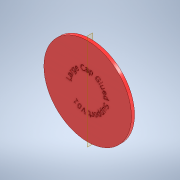
# Autodesk Inventor part: supportForLargeCap
Saved by Autodesk Inventor 2021.1 (Build 251245000, 245)
## iProperties
Created: 2020-09-25
Part Number: supportForLargeCap
Material: PC/ABS Plastic
Document SubType Name: Modeling
Designer: robst
Density: 0.357273 g/cm^3
Appearance: Light Red
Author: robst
Autodesk Inventor part; units mm, degrees
ref_plane "XZ Plane" through (0, 0, 0) normal (0, 1, 0) x (-1, 0, 0)
ref_plane "XY Plane" through (0, 0, 0) normal (0, 0, 1) x (1, 0, 0)
sketch "Sketch1" plane through (0, 0, 0) normal (0, 0, 1) x (1, 0, 0)
  circle A0 centre (0, 0) radius 88.9
  dimension "d0" = 177.8
  constraints: 1 centre point, 1 coincident
  measures "d0" diameter of A0
extrude "Extrusion1" add sketch "Sketch1" against normal blind 6.35
sketch "Sketch2" plane through (0, 0, 0) normal (0, 0, 1) x (1, 0, 0)
  circle A0 centre (0, 0) radius 38.1 construction
  line L0 (-32.4786, 6.8781) -> (-33.0946, 1.0235)
  line L1 (-33.0946, 1.0235) -> (-43.1988, 2.0867)
  line L2 (-43.1988, 2.0867) -> (-43.0575, 3.4296)
  line L3 (-43.0575, 3.4296) -> (-34.1488, 2.4922)
  line L4 (-34.1488, 2.4922) -> (-33.674, 7.0039)
  line L5 (-33.674, 7.0039) -> (-32.4786, 6.8781)
  spline S0 degree 2 poles (-31.6307, 12.0846) (-31.5706, 11.8998) (-31.3457, 11.2701) (-31.3063, 10.9968) knots 0 0 0 1 2 2 2
  spline S1 degree 2 poles (-31.3063, 10.9968) (-31.2407, 10.6193) (-31.2605, 9.958) (-31.442, 9.411) knots 0 0 0 1 2 2 2
  spline S2 degree 2 poles (-31.442, 9.411) (-31.5898, 8.9655) (-32.1928, 8.2721) (-32.5987, 8.0684) knots 0 0 0 1 2 2 2
  spline S3 degree 2 poles (-32.5987, 8.0684) (-32.9915, 7.8778) (-33.9834, 7.8165) (-34.4679, 7.9772) knots 0 0 0 1 2 2 2
  spline S4 degree 2 poles (-34.4679, 7.9772) (-35.2181, 8.2261) (-36.071, 9.2116) (-36.1476, 10.0004) knots 0 0 0 1 2 2 2
  spline S5 degree 2 poles (-36.1476, 10.0004) (-36.2267, 10.7033) (-35.8881, 12.4299) (-35.624, 13.4093) knots 0 0 0 1 2 2 2
  line L6 (-35.624, 13.4093) -> (-35.8584, 13.4871)
  spline S6 degree 2 poles (-35.8584, 13.4871) (-36.2804, 13.627) (-36.8895, 13.5429) (-37.1158, 13.3577) knots 0 0 0 1 2 2 2
  spline S7 degree 2 poles (-37.1158, 13.3577) (-37.342, 13.1725) (-37.6588, 12.5315) (-37.778, 12.1721) knots 0 0 0 1 2 2 2
  spline S8 degree 2 poles (-37.778, 12.1721) (-37.918, 11.7501) (-38.0464, 10.5262) (-37.9934, 9.8753) knots 0 0 0 1 2 2 2
  line L7 (-37.9934, 9.8753) -> (-38.0167, 9.805)
  line L8 (-38.0167, 9.805) -> (-39.2593, 10.2172)
  spline S9 degree 2 poles (-39.2593, 10.2172) (-39.2416, 10.5843) (-39.0586, 11.9203) (-38.8538, 12.5376) knots 0 0 0 1 2 2 2
  spline S10 degree 2 poles (-38.8538, 12.5376) (-38.605, 13.2878) (-38.0309, 14.2338) (-37.5914, 14.539) knots 0 0 0 1 2 2 2
  spline S11 degree 2 poles (-37.5914, 14.539) (-37.1622, 14.8391) (-36.087, 14.9161) (-35.4071, 14.6906) knots 0 0 0 1 2 2 2
  line L9 (-35.4071, 14.6906) -> (-30.4605, 13.0496)
  line L10 (-30.4605, 13.0496) -> (-30.8649, 11.8306)
  line L11 (-30.8649, 11.8306) -> (-31.6307, 12.0846)
  line L12 (-32.6466, 12.4216) -> (-34.655, 13.0878)
  spline S12 degree 2 poles (-34.655, 13.0878) (-34.7611, 12.6373) (-35.0663, 11.2725) (-35.0787, 10.8169) knots 0 0 0 1 2 2 2
  spline S13 degree 2 poles (-35.0787, 10.8169) (-35.0909, 10.2831) (-34.6836, 9.4453) (-34.1365, 9.2639) knots 0 0 0 1 2 2 2
  spline S14 degree 2 poles (-34.1365, 9.2639) (-33.5114, 9.0565) (-32.6451, 9.5498) (-32.4221, 10.2219) knots 0 0 0 1 2 2 2
  spline S15 degree 2 poles (-32.4221, 10.2219) (-32.2329, 10.7923) (-32.4141, 11.8934) (-32.6466, 12.4216) knots 0 0 0 1 2 2 2
  line L13 (-33.1361, 21.2152) -> (-33.1681, 21.1576)
  spline S16 degree 2 poles (-33.1681, 21.1576) (-33.276, 21.0481) (-33.4464, 20.7754) (-33.5543, 20.5811) knots 0 0 0 1 2 2 2
  spline S17 degree 2 poles (-33.5543, 20.5811) (-33.8062, 20.1276) (-33.9062, 19.0152) (-33.7414, 18.3963) knots 0 0 0 1 2 2 2
  line L14 (-33.7414, 18.3963) -> (-29.0128, 15.7693)
  line L15 (-29.0128, 15.7693) -> (-29.6365, 14.6465)
  line L16 (-29.6365, 14.6465) -> (-36.3013, 18.3491)
  line L17 (-36.3013, 18.3491) -> (-35.6775, 19.4718)
  line L18 (-35.6775, 19.4718) -> (-34.6843, 18.9201)
  spline S18 degree 2 poles (-34.6843, 18.9201) (-34.8914, 19.8357) (-34.8298, 20.9977) (-34.5899, 21.4295) knots 0 0 0 1 2 2 2
  spline S19 degree 2 poles (-34.5899, 21.4295) (-34.494, 21.6023) (-34.3836, 21.767) (-34.302, 21.863) knots 0 0 0 1 2 2 2
  line L19 (-34.302, 21.863) -> (-33.1361, 21.2152)
  spline S20 degree 2 poles (-26.0427, 18.4441) (-25.9138, 18.5077) (-25.4518, 18.7753) (-25.1883, 18.9733) knots 0 0 0 1 2 2 2
  spline S21 degree 2 poles (-25.1883, 18.9733) (-24.891, 19.1858) (-24.4221, 19.5767) (-24.1941, 19.8476) knots 0 0 0 1 2 2 2
  spline S22 degree 2 poles (-24.1941, 19.8476) (-23.8124, 20.3011) (-23.5216, 21.1325) (-23.5873, 21.4891) knots 0 0 0 1 2 2 2
  spline S23 degree 2 poles (-23.5873, 21.4891) (-23.6583, 21.8395) (-24.1076, 22.4436) (-24.4666, 22.7458) knots 0 0 0 1 2 2 2
  line L20 (-24.4666, 22.7458) -> (-24.9768, 23.1753)
  spline S24 degree 2 poles (-24.9768, 23.1753) (-24.9644, 22.4868) (-25.2784, 21.449) (-25.7609, 20.8757) knots 0 0 0 1 2 2 2
  spline S25 degree 2 poles (-25.7609, 20.8757) (-26.5986, 19.8805) (-29.0703, 19.9485) (-30.4624, 21.1202) knots 0 0 0 1 2 2 2
  spline S26 degree 2 poles (-30.4624, 21.1202) (-31.1868, 21.7299) (-31.9634, 23.0831) (-32.074, 23.7573) knots 0 0 0 1 2 2 2
  spline S27 degree 2 poles (-32.074, 23.7573) (-32.1699, 24.3977) (-31.8212, 25.6431) (-31.4182, 26.1218) knots 0 0 0 1 2 2 2
  spline S28 degree 2 poles (-31.4182, 26.1218) (-31.0365, 26.5753) (-30.2656, 27.0565) (-29.7893, 27.226) knots 0 0 0 1 2 2 2
  line L21 (-29.7893, 27.226) -> (-29.9873, 27.4894)
  line L22 (-29.9873, 27.4894) -> (-29.2079, 28.4154)
  line L23 (-29.2079, 28.4154) -> (-24.0427, 24.0678)
  spline S29 degree 2 poles (-24.0427, 24.0678) (-22.5561, 22.8166) (-22.2572, 20.3588) (-23.3759, 19.0297) knots 0 0 0 1 2 2 2
  spline S30 degree 2 poles (-23.3759, 19.0297) (-23.7364, 18.6014) (-24.6279, 17.8236) (-25.0647, 17.5347) knots 0 0 0 1 2 2 2
  line L24 (-25.0647, 17.5347) -> (-26.0851, 18.3937)
  line L25 (-26.0851, 18.3937) -> (-26.0427, 18.4441)
  line L26 (-25.7831, 23.8539) -> (-28.9894, 26.5526)
  spline S31 degree 2 poles (-28.9894, 26.5526) (-29.4732, 26.3357) (-30.144, 25.8457) (-30.4038, 25.537) knots 0 0 0 1 2 2 2
  spline S32 degree 2 poles (-30.4038, 25.537) (-31.0294, 24.7937) (-30.6544, 23.0145) (-29.6277, 22.1503) knots 0 0 0 1 2 2 2
  spline S33 degree 2 poles (-29.6277, 22.1503) (-28.6576, 21.3338) (-27.0974, 21.129) (-26.4824, 21.8597) knots 0 0 0 1 2 2 2
  spline S34 degree 2 poles (-26.4824, 21.8597) (-26.159, 22.2439) (-25.7827, 23.3047) (-25.7831, 23.8539) knots 0 0 0 1 2 2 2
  spline S35 degree 2 poles (-19.2664, 26.6093) (-20.7283, 25.5121) (-23.5656, 25.9458) (-24.7024, 27.4604) knots 0 0 0 1 2 2 2
  spline S36 degree 2 poles (-24.7024, 27.4604) (-25.8193, 28.9486) (-25.5833, 31.8847) (-24.3255, 32.8287) knots 0 0 0 1 2 2 2
  spline S37 degree 2 poles (-24.3255, 32.8287) (-23.7592, 33.2537) (-22.6363, 33.5818) (-22.0517, 33.475) knots 0 0 0 1 2 2 2
  spline S38 degree 2 poles (-22.0517, 33.475) (-21.4605, 33.3731) (-20.3553, 32.6275) (-19.8067, 31.8966) knots 0 0 0 1 2 2 2
  line L27 (-19.8067, 31.8966) -> (-19.3866, 31.3369)
  line L28 (-19.3866, 31.3369) -> (-23.6076, 28.1688)
  spline S39 degree 2 poles (-23.6076, 28.1688) (-22.8119, 27.1087) (-20.9, 26.7833) (-19.9517, 27.495) knots 0 0 0 1 2 2 2
  spline S40 degree 2 poles (-19.9517, 27.495) (-19.6159, 27.7471) (-19.0777, 28.3878) (-18.9032, 28.704) knots 0 0 0 1 2 2 2
  spline S41 degree 2 poles (-18.9032, 28.704) (-18.7255, 29.0433) (-18.5165, 29.5604) (-18.4705, 29.7597) knots 0 0 0 1 2 2 2
  line L29 (-18.4705, 29.7597) -> (-18.4112, 29.8042)
  line L30 (-18.4112, 29.8042) -> (-17.571, 28.6847)
  spline S42 degree 2 poles (-17.571, 28.6847) (-17.6945, 28.4789) (-18.0763, 27.8629) (-18.2425, 27.6454) knots 0 0 0 1 2 2 2
  spline S43 degree 2 poles (-18.2425, 27.6454) (-18.4746, 27.3374) (-18.8976, 26.8861) (-19.2664, 26.6093) knots 0 0 0 1 2 2 2
  spline S44 degree 2 poles (-20.9757, 31.3693) (-21.3002, 31.7742) (-21.9261, 32.2516) (-22.2439, 32.3321) knots 0 0 0 1 2 2 2
  spline S45 degree 2 poles (-22.2439, 32.3321) (-22.5947, 32.4292) (-23.3373, 32.2527) (-23.7522, 31.9413) knots 0 0 0 1 2 2 2
  spline S46 degree 2 poles (-23.7522, 31.9413) (-24.1604, 31.6349) (-24.5505, 30.9613) (-24.6096, 30.5463) knots 0 0 0 1 2 2 2
  spline S47 degree 2 poles (-24.6096, 30.5463) (-24.6572, 30.1297) (-24.4544, 29.3657) (-24.1957, 28.9525) knots 0 0 0 1 2 2 2
  line L31 (-24.1957, 28.9525) -> (-20.9757, 31.3693)
  spline S48 degree 2 poles (-8.1335, 31.8258) (-9.0845, 31.5578) (-10.8741, 31.7464) (-11.6414, 32.2231) knots 0 0 0 1 2 2 2
  spline S49 degree 2 poles (-11.6414, 32.2231) (-12.4065, 32.6919) (-13.5843, 34.4129) (-13.9327, 35.6492) knots 0 0 0 1 2 2 2
  spline S50 degree 2 poles (-13.9327, 35.6492) (-14.2788, 36.8776) (-14.1663, 38.8767) (-13.7618, 39.7177) knots 0 0 0 1 2 2 2
  spline S51 degree 2 poles (-13.7618, 39.7177) (-13.3607, 40.5407) (-11.9541, 41.6813) (-10.9635, 41.9604) knots 0 0 0 1 2 2 2
  spline S52 degree 2 poles (-10.9635, 41.9604) (-10.4722, 42.0988) (-9.5682, 42.1996) (-9.1724, 42.1913) knots 0 0 0 1 2 2 2
  spline S53 degree 2 poles (-9.1724, 42.1913) (-8.8264, 42.1776) (-8.086, 42.0698) (-7.7119, 41.987) knots 0 0 0 1 2 2 2
  line L32 (-7.7119, 41.987) -> (-7.2698, 40.4179)
  line L33 (-7.2698, 40.4179) -> (-7.3728, 40.3888)
  spline S54 degree 2 poles (-7.3728, 40.3888) (-7.5918, 40.4982) (-8.2558, 40.7901) (-8.7044, 40.8947) knots 0 0 0 1 2 2 2
  spline S55 degree 2 poles (-8.7044, 40.8947) (-9.1349, 40.9958) (-10.0882, 41.0095) (-10.6588, 40.8487) knots 0 0 0 1 2 2 2
  spline S56 degree 2 poles (-10.6588, 40.8487) (-11.2849, 40.6723) (-12.2571, 39.8423) (-12.5387, 39.2326) knots 0 0 0 1 2 2 2
  spline S57 degree 2 poles (-12.5387, 39.2326) (-12.8101, 38.6173) (-12.8433, 36.9741) (-12.5775, 36.0311) knots 0 0 0 1 2 2 2
  spline S58 degree 2 poles (-12.5775, 36.0311) (-12.2939, 35.0246) (-11.4019, 33.7106) (-10.8412, 33.3297) knots 0 0 0 1 2 2 2
  spline S59 degree 2 poles (-10.8412, 33.3297) (-10.2929, 32.9624) (-9.0529, 32.7814) (-8.4348, 32.9556) knots 0 0 0 1 2 2 2
  spline S60 degree 2 poles (-8.4348, 32.9556) (-7.8721, 33.1141) (-6.9914, 33.6617) (-6.677, 33.9727) knots 0 0 0 1 2 2 2
  spline S61 degree 2 poles (-6.677, 33.9727) (-6.3784, 34.2792) (-5.968, 34.8567) (-5.8599, 35.0497) knots 0 0 0 1 2 2 2
  line L34 (-5.8599, 35.0497) -> (-5.7648, 35.0765)
  line L35 (-5.7648, 35.0765) -> (-5.3271, 33.5233)
  spline S62 degree 2 poles (-5.3271, 33.5233) (-5.6096, 33.2812) (-6.102, 32.843) (-6.4705, 32.6023) knots 0 0 0 1 2 2 2
  spline S63 degree 2 poles (-6.4705, 32.6023) (-6.8582, 32.3391) (-7.5471, 31.991) (-8.1335, 31.8258) knots 0 0 0 1 2 2 2
  spline S64 degree 2 poles (0.2363, 33.8598) (0.0843, 33.7387) (-0.4267, 33.3075) (-0.6689, 33.1748) knots 0 0 0 1 2 2 2
  spline S65 degree 2 poles (-0.6689, 33.1748) (-0.9994, 32.9811) (-1.6258, 32.768) (-2.2018, 32.7463) knots 0 0 0 1 2 2 2
  spline S66 degree 2 poles (-2.2018, 32.7463) (-2.6707, 32.7286) (-3.5315, 33.0504) (-3.8645, 33.3592) knots 0 0 0 1 2 2 2
  spline S67 degree 2 poles (-3.8645, 33.3592) (-4.1807, 33.6604) (-4.5856, 34.568) (-4.6048, 35.0781) knots 0 0 0 1 2 2 2
  spline S68 degree 2 poles (-4.6048, 35.0781) (-4.6346, 35.8679) (-4.0103, 37.012) (-3.2984, 37.3601) knots 0 0 0 1 2 2 2
  spline S69 degree 2 poles (-3.2984, 37.3601) (-2.6678, 37.6805) (-0.9319, 37.9683) (0.0779, 38.064) knots 0 0 0 1 2 2 2
  line L36 (0.0779, 38.064) -> (0.0686, 38.3109)
  spline S70 degree 2 poles (0.0686, 38.3109) (0.0519, 38.7552) (-0.2404, 39.2962) (-0.4931, 39.4432) knots 0 0 0 1 2 2 2
  spline S71 degree 2 poles (-0.4931, 39.4432) (-0.7458, 39.5902) (-1.4571, 39.6623) (-1.8356, 39.648) knots 0 0 0 1 2 2 2
  spline S72 degree 2 poles (-1.8356, 39.648) (-2.2799, 39.6313) (-3.4712, 39.3228) (-4.0622, 39.0451) knots 0 0 0 1 2 2 2
  line L37 (-4.0622, 39.0451) -> (-4.1362, 39.0423)
  line L38 (-4.1362, 39.0423) -> (-4.1855, 40.3505)
  spline S73 degree 2 poles (-4.1855, 40.3505) (-3.8354, 40.4625) (-2.5201, 40.7593) (-1.8701, 40.7838) knots 0 0 0 1 2 2 2
  spline S74 degree 2 poles (-1.8701, 40.7838) (-1.0803, 40.8135) (0.0068, 40.6073) (0.4467, 40.3025) knots 0 0 0 1 2 2 2
  spline S75 degree 2 poles (0.4467, 40.3025) (0.8781, 40.0057) (1.327, 39.0257) (1.354, 38.3099) knots 0 0 0 1 2 2 2
  line L39 (1.354, 38.3099) -> (1.5502, 33.1018)
  line L40 (1.5502, 33.1018) -> (0.2667, 33.0535)
  line L41 (0.2667, 33.0535) -> (0.2363, 33.8598)
  line L42 (0.196, 34.9294) -> (0.1163, 37.0438)
  spline S76 degree 2 poles (0.1163, 37.0438) (-0.3428, 36.9853) (-1.728, 36.7931) (-2.1591, 36.645) knots 0 0 0 1 2 2 2
  spline S77 degree 2 poles (-2.1591, 36.645) (-2.6634, 36.4695) (-3.3053, 35.7944) (-3.2836, 35.2185) knots 0 0 0 1 2 2 2
  spline S78 degree 2 poles (-3.2836, 35.2185) (-3.2588, 34.5603) (-2.4932, 33.9217) (-1.7856, 33.9484) knots 0 0 0 1 2 2 2
  spline S79 degree 2 poles (-1.7856, 33.9484) (-1.185, 33.971) (-0.2173, 34.5265) (0.196, 34.9294) knots 0 0 0 1 2 2 2
  spline S80 degree 2 poles (10.3689, 35.7246) (10.0093, 33.8486) (7.7976, 31.9756) (6.431, 32.2375) knots 0 0 0 1 2 2 2
  spline S81 degree 2 poles (6.431, 32.2375) (5.873, 32.3445) (5.0655, 32.7675) (4.6719, 33.1196) knots 0 0 0 1 2 2 2
  line L43 (4.6719, 33.1196) -> (4.0705, 29.9822)
  line L44 (4.0705, 29.9822) -> (2.8091, 30.224)
  line L45 (2.8091, 30.224) -> (4.7729, 40.4692)
  line L46 (4.7729, 40.4692) -> (6.0344, 40.2274)
  line L47 (6.0344, 40.2274) -> (5.884, 39.443)
  spline S82 degree 2 poles (5.884, 39.443) (6.4352, 39.7817) (7.6919, 40.1276) (8.3631, 39.999) knots 0 0 0 1 2 2 2
  spline S83 degree 2 poles (8.3631, 39.999) (9.6488, 39.7525) (10.6975, 37.4389) (10.3689, 35.7246) knots 0 0 0 1 2 2 2
  spline S84 degree 2 poles (9.0391, 35.8286) (9.2856, 37.1143) (8.7401, 38.686) (7.8264, 38.8611) knots 0 0 0 1 2 2 2
  spline S85 degree 2 poles (7.8264, 38.8611) (7.2927, 38.9634) (6.1986, 38.6785) (5.6825, 38.3918) knots 0 0 0 1 2 2 2
  line L48 (5.6825, 38.3918) -> (4.8672, 34.1385)
  spline S86 degree 2 poles (4.8672, 34.1385) (5.3155, 33.8094) (5.9849, 33.4967) (6.4378, 33.4099) knots 0 0 0 1 2 2 2
  spline S87 degree 2 poles (6.4378, 33.4099) (7.4162, 33.2223) (8.7756, 34.454) (9.0391, 35.8286) knots 0 0 0 1 2 2 2
  spline S88 degree 2 poles (18.4556, 27.1493) (17.5523, 27.7387) (16.4159, 29.2666) (16.2424, 30.1761) knots 0 0 0 1 2 2 2
  spline S89 degree 2 poles (16.2424, 30.1761) (16.0735, 31.0924) (16.5899, 33.1345) (17.2963, 34.2171) knots 0 0 0 1 2 2 2
  spline S90 degree 2 poles (17.2963, 34.2171) (17.9666, 35.2446) (19.6076, 36.494) (20.5233, 36.7223) knots 0 0 0 1 2 2 2
  spline S91 degree 2 poles (20.5233, 36.7223) (21.4049, 36.9434) (23.3178, 36.5605) (24.2211, 35.9711) knots 0 0 0 1 2 2 2
  spline S92 degree 2 poles (24.2211, 35.9711) (24.6556, 35.6877) (25.3607, 35.0507) (25.6473, 34.7064) knots 0 0 0 1 2 2 2
  spline S93 degree 2 poles (25.6473, 34.7064) (25.8829, 34.4347) (26.3883, 33.6724) (26.53, 33.4226) knots 0 0 0 1 2 2 2
  line L49 (26.53, 33.4226) -> (25.6393, 32.0573)
  line L50 (25.6393, 32.0573) -> (25.5427, 32.1203)
  spline S94 degree 2 poles (25.5427, 32.1203) (25.4504, 32.4459) (25.2227, 33.0762) (24.9349, 33.5393) knots 0 0 0 1 2 2 2
  spline S95 degree 2 poles (24.9349, 33.5393) (24.7026, 33.9366) (23.9615, 34.7445) (23.4513, 35.0774) knots 0 0 0 1 2 2 2
  spline S96 degree 2 poles (23.4513, 35.0774) (22.2239, 35.8782) (19.5011, 35.02) (18.4979, 33.4823) knots 0 0 0 1 2 2 2
  spline S97 degree 2 poles (18.4979, 33.4823) (17.94, 32.6273) (17.5032, 31.0838) (17.5945, 30.395) knots 0 0 0 1 2 2 2
  spline S98 degree 2 poles (17.5945, 30.395) (17.672, 29.7152) (18.4049, 28.5784) (19.0531, 28.1555) knots 0 0 0 1 2 2 2
  spline S99 degree 2 poles (19.0531, 28.1555) (19.5289, 27.8451) (20.5704, 27.3621) (20.9845, 27.2886) knots 0 0 0 1 2 2 2
  line L51 (20.9845, 27.2886) -> (22.4197, 29.4883)
  line L52 (22.4197, 29.4883) -> (20.4475, 30.775)
  line L53 (20.4475, 30.775) -> (21.0954, 31.7679)
  line L54 (21.0954, 31.7679) -> (24.1846, 29.7524)
  line L55 (24.1846, 29.7524) -> (21.7597, 26.0357)
  spline S100 degree 2 poles (21.7597, 26.0357) (21.4829, 26.0786) (20.5585, 26.259) (20.1898, 26.3718) knots 0 0 0 1 2 2 2
  spline S101 degree 2 poles (20.1898, 26.3718) (19.6881, 26.5221) (18.9314, 26.8389) (18.4556, 27.1493) knots 0 0 0 1 2 2 2
  line L56 (23.3718, 23.3344) -> (22.4468, 24.2255)
  line L57 (22.4468, 24.2255) -> (29.8099, 31.8685)
  line L58 (29.8099, 31.8685) -> (30.7349, 30.9774)
  line L59 (30.7349, 30.9774) -> (23.3718, 23.3344)
  line L60 (28.2845, 17.2942) -> (27.5192, 18.3257)
  line L61 (27.5192, 18.3257) -> (28.1937, 18.8261)
  spline S102 degree 2 poles (28.1937, 18.8261) (27.4239, 18.9931) (26.3613, 19.5273) (25.9688, 20.0562) knots 0 0 0 1 2 2 2
  spline S103 degree 2 poles (25.9688, 20.0562) (25.6745, 20.453) (25.414, 21.3567) (25.507, 21.8255) knots 0 0 0 1 2 2 2
  spline S104 degree 2 poles (25.507, 21.8255) (25.5951, 22.301) (26.2455, 23.2346) (26.867, 23.6957) knots 0 0 0 1 2 2 2
  line L62 (26.867, 23.6957) -> (30.841, 26.6441)
  line L63 (30.841, 26.6441) -> (31.6063, 25.6126)
  line L64 (31.6063, 25.6126) -> (28.115, 23.0223)
  spline S105 degree 2 poles (28.115, 23.0223) (27.6257, 22.6593) (27.0383, 22.1107) (26.8935, 21.8085) knots 0 0 0 1 2 2 2
  spline S106 degree 2 poles (26.8935, 21.8085) (26.7486, 21.5062) (26.8493, 20.9145) (27.1486, 20.5112) knots 0 0 0 1 2 2 2
  spline S107 degree 2 poles (27.1486, 20.5112) (27.4282, 20.1343) (28.4908, 19.6002) (29.0665, 19.4737) knots 0 0 0 1 2 2 2
  line L65 (29.0665, 19.4737) -> (33.6422, 22.8685)
  line L66 (33.6422, 22.8685) -> (34.4075, 21.837)
  line L67 (34.4075, 21.837) -> (28.2845, 17.2942)
  spline S108 degree 2 poles (30.3491, 12.577) (29.6205, 14.2533) (30.6998, 16.913) (32.4365, 17.6679) knots 0 0 0 1 2 2 2
  spline S109 degree 2 poles (32.4365, 17.6679) (34.143, 18.4097) (36.9445, 17.4998) (37.5714, 16.0575) knots 0 0 0 1 2 2 2
  spline S110 degree 2 poles (37.5714, 16.0575) (37.8537, 15.4082) (37.9126, 14.2398) (37.6733, 13.6958) knots 0 0 0 1 2 2 2
  spline S111 degree 2 poles (37.6733, 13.6958) (37.4372, 13.1443) (36.4559, 12.242) (35.6177, 11.8776) knots 0 0 0 1 2 2 2
  line L68 (35.6177, 11.8776) -> (34.9759, 11.5987)
  line L69 (34.9759, 11.5987) -> (32.872, 16.4388)
  spline S112 degree 2 poles (32.872, 16.4388) (31.6563, 15.9103) (30.8968, 14.1258) (31.3695, 13.0385) knots 0 0 0 1 2 2 2
  spline S113 degree 2 poles (31.3695, 13.0385) (31.5368, 12.6534) (32.0355, 11.9814) (32.3027, 11.7384) knots 0 0 0 1 2 2 2
  spline S114 degree 2 poles (32.3027, 11.7384) (32.5915, 11.4869) (33.0462, 11.1639) (33.2294, 11.0729) knots 0 0 0 1 2 2 2
  line L70 (33.2294, 11.0729) -> (33.2589, 11.0049)
  line L71 (33.2589, 11.0049) -> (31.9752, 10.447)
  spline S115 degree 2 poles (31.9752, 10.447) (31.8036, 10.6147) (31.2928, 11.1289) (31.1198, 11.341) knots 0 0 0 1 2 2 2
  spline S116 degree 2 poles (31.1198, 11.341) (30.8739, 11.6381) (30.5329, 12.1542) (30.3491, 12.577) knots 0 0 0 1 2 2 2
  spline S117 degree 2 poles (35.3755, 13.137) (35.8447, 13.3589) (36.454, 13.8571) (36.6061, 14.1477) knots 0 0 0 1 2 2 2
  spline S118 degree 2 poles (36.6061, 14.1477) (36.7817, 14.4664) (36.7821, 15.2297) (36.5753, 15.7054) knots 0 0 0 1 2 2 2
  spline S119 degree 2 poles (36.5753, 15.7054) (36.3718, 16.1735) (35.8069, 16.709) (35.4169, 16.8627) knots 0 0 0 1 2 2 2
  spline S120 degree 2 poles (35.4169, 16.8627) (35.0227, 17.0055) (34.2325, 16.9853) (33.7706, 16.8294) knots 0 0 0 1 2 2 2
  line L72 (33.7706, 16.8294) -> (35.3755, 13.137)
  line L73 (33.0028, 3.1185) -> (32.7694, 4.3815)
  line L74 (32.7694, 4.3815) -> (33.5305, 4.5222)
  spline S121 degree 2 poles (33.5305, 4.5222) (33.2337, 4.7687) (32.8306, 5.138) (32.6391, 5.404) knots 0 0 0 1 2 2 2
  spline S122 degree 2 poles (32.6391, 5.404) (32.4601, 5.6473) (32.2163, 6.1967) (32.1459, 6.5772) knots 0 0 0 1 2 2 2
  spline S123 degree 2 poles (32.1459, 6.5772) (32.0322, 7.1925) (32.3508, 8.3231) (32.7773, 8.7787) knots 0 0 0 1 2 2 2
  spline S124 degree 2 poles (32.7773, 8.7787) (33.2039, 9.2343) (34.5864, 9.9084) (35.5336, 10.0835) knots 0 0 0 1 2 2 2
  spline S125 degree 2 poles (35.5336, 10.0835) (36.5214, 10.266) (38.0568, 10.0223) (38.6815, 9.6773) knots 0 0 0 1 2 2 2
  spline S126 degree 2 poles (38.6815, 9.6773) (39.2436, 9.3541) (40.0162, 8.2996) (40.1344, 7.66) knots 0 0 0 1 2 2 2
  spline S127 degree 2 poles (40.1344, 7.66) (40.2377, 7.1014) (40.1408, 6.2211) (39.967, 5.7117) knots 0 0 0 1 2 2 2
  line L75 (39.967, 5.7117) -> (43.2055, 6.3102)
  line L76 (43.2055, 6.3102) -> (43.4389, 5.0472)
  line L77 (43.4389, 5.0472) -> (33.0028, 3.1185)
  line L78 (34.5911, 4.7182) -> (38.9226, 5.5187)
  spline S128 degree 2 poles (38.9226, 5.5187) (39.0625, 6.0301) (39.0949, 6.8064) (39.0156, 7.2355) knots 0 0 0 1 2 2 2
  spline S129 degree 2 poles (39.0156, 7.2355) (38.836, 8.2071) (37.1752, 9.0389) (35.7988, 8.7845) knots 0 0 0 1 2 2 2
  spline S130 degree 2 poles (35.7988, 8.7845) (34.471, 8.5391) (33.226, 7.4382) (33.3981, 6.5072) knots 0 0 0 1 2 2 2
  spline S131 degree 2 poles (33.3981, 6.5072) (33.4893, 6.0133) (34.1283, 5.0931) (34.5911, 4.7182) knots 0 0 0 1 2 2 2
  spline S132 degree 2 poles (32.2963, -5.9446) (32.497, -4.8597) (33.2319, -3.4215) (33.6801, -2.8095) knots 0 0 0 1 2 2 2
  line L79 (33.6801, -2.8095) -> (35.3479, -3.1179)
  line L80 (35.3479, -3.1179) -> (35.3299, -3.2151)
  spline S133 degree 2 poles (35.3299, -3.2151) (34.5933, -3.7571) (33.6062, -5.291) (33.464, -6.0601) knots 0 0 0 1 2 2 2
  spline S134 degree 2 poles (33.464, -6.0601) (33.2603, -7.1611) (33.967, -8.4557) (34.7199, -8.595) knots 0 0 0 1 2 2 2
  spline S135 degree 2 poles (34.7199, -8.595) (35.319, -8.7058) (36.1732, -8.2526) (36.4777, -7.6474) knots 0 0 0 1 2 2 2
  spline S136 degree 2 poles (36.4777, -7.6474) (36.6926, -7.2099) (37.013, -6.4737) (37.265, -5.9259) knots 0 0 0 1 2 2 2
  spline S137 degree 2 poles (37.265, -5.9259) (37.4985, -5.4332) (38.0627, -4.6919) (38.453, -4.4375) knots 0 0 0 1 2 2 2
  spline S138 degree 2 poles (38.453, -4.4375) (38.8418, -4.1913) (39.7953, -4.016) (40.3782, -4.1238) knots 0 0 0 1 2 2 2
  spline S139 degree 2 poles (40.3782, -4.1238) (41.5926, -4.3484) (42.8857, -6.5469) (42.6146, -8.0123) knots 0 0 0 1 2 2 2
  spline S140 degree 2 poles (42.6146, -8.0123) (42.4589, -8.8543) (41.8514, -10.2825) (41.4174, -10.8637) knots 0 0 0 1 2 2 2
  line L81 (41.4174, -10.8637) -> (39.8305, -10.5702)
  line L82 (39.8305, -10.5702) -> (39.8485, -10.473)
  spline S141 degree 2 poles (39.8485, -10.473) (40.374, -10.0762) (41.2973, -8.7064) (41.4485, -7.8887) knots 0 0 0 1 2 2 2
  spline S142 degree 2 poles (41.4485, -7.8887) (41.6193, -6.9657) (40.9641, -5.6639) (40.2598, -5.5337) knots 0 0 0 1 2 2 2
  spline S143 degree 2 poles (40.2598, -5.5337) (39.6283, -5.4168) (38.751, -5.9495) (38.4642, -6.5496) knots 0 0 0 1 2 2 2
  spline S144 degree 2 poles (38.4642, -6.5496) (38.273, -6.9496) (37.7554, -8.1182) (37.5591, -8.5006) knots 0 0 0 1 2 2 2
  spline S145 degree 2 poles (37.5591, -8.5006) (37.0532, -9.4703) (35.6054, -10.1906) (34.6743, -10.0184) knots 0 0 0 1 2 2 2
  spline S146 degree 2 poles (34.6743, -10.0184) (34.0833, -9.909) (33.0382, -9.2217) (32.7209, -8.7192) knots 0 0 0 1 2 2 2
  spline S147 degree 2 poles (32.7209, -8.7192) (32.3721, -8.1607) (32.1271, -6.8594) (32.2963, -5.9446) knots 0 0 0 1 2 2 2
  line L83 (28.9807, -16.1005) -> (29.5016, -14.9265)
  line L84 (29.5016, -14.9265) -> (30.2692, -15.267)
  spline S148 degree 2 poles (30.2692, -15.267) (30.0355, -14.5148) (29.977, -13.3269) (30.2442, -12.7248) knots 0 0 0 1 2 2 2
  spline S149 degree 2 poles (30.2442, -12.7248) (30.4445, -12.2733) (31.1028, -11.6016) (31.5567, -11.4516) knots 0 0 0 1 2 2 2
  spline S150 degree 2 poles (31.5567, -11.4516) (32.0138, -11.2942) (33.1466, -11.4005) (33.8541, -11.7143) knots 0 0 0 1 2 2 2
  line L85 (33.8541, -11.7143) -> (38.3772, -13.7211)
  line L86 (38.3772, -13.7211) -> (37.8563, -14.8951)
  line L87 (37.8563, -14.8951) -> (33.8826, -13.1321)
  spline S151 degree 2 poles (33.8826, -13.1321) (33.3257, -12.885) (32.5589, -12.6439) (32.2245, -12.6667) knots 0 0 0 1 2 2 2
  spline S152 degree 2 poles (32.2245, -12.6667) (31.8902, -12.6895) (31.4248, -13.0685) (31.2211, -13.5276) knots 0 0 0 1 2 2 2
  spline S153 degree 2 poles (31.2211, -13.5276) (31.0308, -13.9566) (31.0892, -15.1444) (31.2626, -15.7078) knots 0 0 0 1 2 2 2
  line L88 (31.2626, -15.7078) -> (36.4706, -18.0184)
  line L89 (36.4706, -18.0184) -> (35.9497, -19.1924)
  line L90 (35.9497, -19.1924) -> (28.9807, -16.1005)
  spline S154 degree 2 poles (27.3575, -25.2057) (25.8385, -24.0476) (25.1477, -21.2329) (25.9913, -20.1263) knots 0 0 0 1 2 2 2
  spline S155 degree 2 poles (25.9913, -20.1263) (26.3357, -19.6746) (27.0744, -19.1403) (27.565, -18.9449) knots 0 0 0 1 2 2 2
  line L91 (27.565, -18.9449) -> (25.0246, -17.008)
  line L92 (25.0246, -17.008) -> (25.8033, -15.9866)
  line L93 (25.8033, -15.9866) -> (34.099, -22.3113)
  line L94 (34.099, -22.3113) -> (33.3203, -23.3327)
  line L95 (33.3203, -23.3327) -> (32.6852, -22.8485)
  spline S156 degree 2 poles (32.6852, -22.8485) (32.7427, -23.4928) (32.4922, -24.772) (32.0778, -25.3154) knots 0 0 0 1 2 2 2
  spline S157 degree 2 poles (32.0778, -25.3154) (31.2841, -26.3565) (28.7456, -26.264) (27.3575, -25.2057) knots 0 0 0 1 2 2 2
  spline S158 degree 2 poles (28.0434, -24.0617) (29.0844, -24.8554) (30.7344, -25.0677) (31.2985, -24.3278) knots 0 0 0 1 2 2 2
  spline S159 degree 2 poles (31.2985, -24.3278) (31.6279, -23.8957) (31.8606, -22.7893) (31.834, -22.1995) knots 0 0 0 1 2 2 2
  line L96 (31.834, -22.1995) -> (28.39, -19.5738)
  spline S160 degree 2 poles (28.39, -19.5738) (27.8956, -19.8285) (27.3173, -20.2883) (27.0377, -20.655) knots 0 0 0 1 2 2 2
  spline S161 degree 2 poles (27.0377, -20.655) (26.4337, -21.4472) (26.9303, -23.2131) (28.0434, -24.0617) knots 0 0 0 1 2 2 2
  spline S162 degree 2 poles (20.8036, -30.8379) (19.5928, -29.3605) (19.57, -26.4623) (20.6462, -25.5803) knots 0 0 0 1 2 2 2
  spline S163 degree 2 poles (20.6462, -25.5803) (21.0856, -25.2201) (21.9276, -24.8707) (22.4501, -24.7938) knots 0 0 0 1 2 2 2
  line L97 (22.4501, -24.7938) -> (20.4251, -22.3231)
  line L98 (20.4251, -22.3231) -> (21.4184, -21.5089)
  line L99 (21.4184, -21.5089) -> (28.031, -29.577)
  line L100 (28.031, -29.577) -> (27.0377, -30.3911)
  line L101 (27.0377, -30.3911) -> (26.5314, -29.7735)
  spline S164 degree 2 poles (26.5314, -29.7735) (26.4387, -30.4137) (25.8998, -31.6005) (25.3712, -32.0337) knots 0 0 0 1 2 2 2
  spline S165 degree 2 poles (25.3712, -32.0337) (24.3588, -32.8635) (21.9101, -32.1878) (20.8036, -30.8379) knots 0 0 0 1 2 2 2
  spline S166 degree 2 poles (21.7349, -29.883) (22.5647, -30.8954) (24.1212, -31.4827) (24.8408, -30.8929) knots 0 0 0 1 2 2 2
  spline S167 degree 2 poles (24.8408, -30.8929) (25.2611, -30.5485) (25.7428, -29.5256) (25.8529, -28.9456) knots 0 0 0 1 2 2 2
  line L102 (25.8529, -28.9456) -> (23.1077, -25.5961)
  spline S168 degree 2 poles (23.1077, -25.5961) (22.5679, -25.7298) (21.8991, -26.0438) (21.5425, -26.3361) knots 0 0 0 1 2 2 2
  spline S169 degree 2 poles (21.5425, -26.3361) (20.7719, -26.9676) (20.8476, -28.8004) (21.7349, -29.883) knots 0 0 0 1 2 2 2
  spline S170 degree 2 poles (13.1572, -34.5699) (12.3091, -32.84) (13.0482, -30.1394) (14.4381, -29.458) knots 0 0 0 1 2 2 2
  spline S171 degree 2 poles (14.4381, -29.458) (15.8648, -28.7584) (18.4519, -29.9017) (19.271, -31.5725) knots 0 0 0 1 2 2 2
  spline S172 degree 2 poles (19.271, -31.5725) (20.1119, -33.2876) (19.3578, -36.0139) (17.9828, -36.688) knots 0 0 0 1 2 2 2
  spline S173 degree 2 poles (17.9828, -36.688) (16.593, -37.3694) (14.0018, -36.2924) (13.1572, -34.5699) knots 0 0 0 1 2 2 2
  spline S174 degree 2 poles (14.3475, -33.9864) (14.9999, -35.317) (16.6026, -36.136) (17.4971, -35.6974) knots 0 0 0 1 2 2 2
  spline S175 degree 2 poles (17.4971, -35.6974) (18.3916, -35.2588) (18.7332, -33.4867) (18.0808, -32.156) knots 0 0 0 1 2 2 2
  spline S176 degree 2 poles (18.0808, -32.156) (17.4465, -30.8623) (15.8183, -30.01) (14.9237, -30.4486) knots 0 0 0 1 2 2 2
  spline S177 degree 2 poles (14.9237, -30.4486) (14.0366, -30.8835) (13.7023, -32.6705) (14.3475, -33.9864) knots 0 0 0 1 2 2 2
  line L103 (7.9312, -38.5381) -> (7.9947, -38.5208)
  spline S178 degree 2 poles (7.9947, -38.5208) (8.1485, -38.5216) (8.4627, -38.4533) (8.6772, -38.395) knots 0 0 0 1 2 2 2
  spline S179 degree 2 poles (8.6772, -38.395) (9.1778, -38.259) (10.0442, -37.5542) (10.3725, -37.0043) knots 0 0 0 1 2 2 2
  line L104 (10.3725, -37.0043) -> (8.9539, -31.7843)
  line L105 (8.9539, -31.7843) -> (10.1933, -31.4474)
  line L106 (10.1933, -31.4474) -> (12.1929, -38.8047)
  line L107 (12.1929, -38.8047) -> (10.9534, -39.1415)
  line L108 (10.9534, -39.1415) -> (10.6554, -38.0451)
  spline S180 degree 2 poles (10.6554, -38.0451) (10.1442, -38.8325) (9.269, -39.5993) (8.7923, -39.7289) knots 0 0 0 1 2 2 2
  spline S181 degree 2 poles (8.7923, -39.7289) (8.6016, -39.7807) (8.4066, -39.8166) (8.281, -39.8252) knots 0 0 0 1 2 2 2
  line L109 (8.281, -39.8252) -> (7.9312, -38.5381)
  spline S182 degree 2 poles (2.9956, -32.7473) (4.0339, -32.6237) (5.3442, -33.6699) (5.4971, -34.9535) knots 0 0 0 1 2 2 2
  line L110 (5.4971, -34.9535) -> (5.9965, -39.1476)
  line L111 (5.9965, -39.1476) -> (6.8549, -39.0454)
  line L112 (6.8549, -39.0454) -> (6.9805, -40.1)
  line L113 (6.9805, -40.1) -> (6.1221, -40.2023)
  line L114 (6.1221, -40.2023) -> (6.381, -42.377)
  line L115 (6.381, -42.377) -> (5.1056, -42.5288)
  line L116 (5.1056, -42.5288) -> (4.8467, -40.3541)
  line L117 (4.8467, -40.3541) -> (2.5003, -40.6335)
  line L118 (2.5003, -40.6335) -> (2.3747, -39.5789)
  line L119 (2.3747, -39.5789) -> (4.7211, -39.2995)
  line L120 (4.7211, -39.2995) -> (4.2918, -35.694)
  spline S183 degree 2 poles (4.2918, -35.694) (4.2236, -35.1217) (4.1078, -34.4971) (3.9367, -34.2438) knots 0 0 0 1 2 2 2
  spline S184 degree 2 poles (3.9367, -34.2438) (3.794, -34.0204) (3.2507, -33.8446) (2.8092, -33.8972) knots 0 0 0 1 2 2 2
  spline S185 degree 2 poles (2.8092, -33.8972) (2.4985, -33.9342) (1.9404, -34.1913) (1.8164, -34.2641) knots 0 0 0 1 2 2 2
  line L121 (1.8164, -34.2641) -> (1.7429, -34.2729)
  line L122 (1.7429, -34.2729) -> (1.6066, -33.1283)
  spline S186 degree 2 poles (1.6066, -33.1283) (1.9546, -32.9874) (2.6768, -32.7853) (2.9956, -32.7473) knots 0 0 0 1 2 2 2
  line L123 (-13.1413, -41.3426) -> (-7.5874, -32.1435)
  line L124 (-7.5874, -32.1435) -> (-6.1625, -32.4494)
  line L125 (-6.1625, -32.4494) -> (-4.874, -43.1175)
  line L126 (-4.874, -43.1175) -> (-6.2908, -42.8134)
  line L127 (-6.2908, -42.8134) -> (-7.2724, -33.9711)
  line L128 (-7.2724, -33.9711) -> (-11.797, -41.6312)
  line L129 (-11.797, -41.6312) -> (-13.1413, -41.3426)
  spline S187 degree 2 poles (-19.6245, -32.8187) (-18.4262, -30.3618) (-15.8755, -28.757) (-14.3881, -29.4824) knots 0 0 0 1 2 2 2
  spline S188 degree 2 poles (-14.3881, -29.4824) (-12.8785, -30.2187) (-12.6091, -33.2539) (-13.7821, -35.6589) knots 0 0 0 1 2 2 2
  spline S189 degree 2 poles (-13.7821, -35.6589) (-14.9876, -38.1306) (-17.531, -39.7207) (-19.0259, -38.9916) knots 0 0 0 1 2 2 2
  spline S190 degree 2 poles (-19.0259, -38.9916) (-20.5281, -38.259) (-20.7866, -35.2016) (-19.6245, -32.8187) knots 0 0 0 1 2 2 2
  spline S191 degree 2 poles (-16.6986, -30.8014) (-17.0963, -31.1662) (-17.9229, -32.4852) (-18.3812, -33.425) knots 0 0 0 1 2 2 2
  spline S192 degree 2 poles (-18.3812, -33.425) (-18.8396, -34.3649) (-19.3665, -35.8209) (-19.4089, -36.3773) knots 0 0 0 1 2 2 2
  spline S193 degree 2 poles (-19.4089, -36.3773) (-19.4513, -36.9338) (-19.042, -37.7288) (-18.5314, -37.9778) knots 0 0 0 1 2 2 2
  spline S194 degree 2 poles (-18.5314, -37.9778) (-18.0208, -38.2268) (-17.1276, -38.067) (-16.7006, -37.6799) knots 0 0 0 1 2 2 2
  spline S195 degree 2 poles (-16.7006, -37.6799) (-16.2882, -37.3039) (-15.4621, -35.948) (-15.0253, -35.0526) knots 0 0 0 1 2 2 2
  spline S196 degree 2 poles (-15.0253, -35.0526) (-14.5562, -34.0906) (-14.0466, -32.7452) (-13.9935, -32.1481) knots 0 0 0 1 2 2 2
  spline S197 degree 2 poles (-13.9935, -32.1481) (-13.9402, -31.5879) (-14.3497, -30.7561) (-14.8826, -30.4962) knots 0 0 0 1 2 2 2
  spline S198 degree 2 poles (-14.8826, -30.4962) (-15.3858, -30.2508) (-16.279, -30.4106) (-16.6986, -30.8014) knots 0 0 0 1 2 2 2
  line L130 (-22.9371, -23.9042) -> (-19.0945, -27.0349)
  line L131 (-19.0945, -27.0349) -> (-19.7497, -27.8392)
  line L132 (-19.7497, -27.8392) -> (-21.1795, -26.6743)
  line L133 (-21.1795, -26.6743) -> (-25.4803, -31.9531)
  line L134 (-25.4803, -31.9531) -> (-24.0505, -33.118)
  line L135 (-24.0505, -33.118) -> (-24.6381, -33.8393)
  spline S199 degree 2 poles (-24.6381, -33.8393) (-25.4488, -33.1789) (-26.5892, -33.0144) (-27.1603, -33.6111) knots 0 0 0 1 2 2 2
  line L136 (-27.1603, -33.6111) -> (-27.9773, -32.9455)
  line L137 (-27.9773, -32.9455) -> (-22.1945, -25.8474)
  line L138 (-22.1945, -25.8474) -> (-23.5924, -24.7085)
  line L139 (-23.5924, -24.7085) -> (-22.9371, -23.9042)
  dimension "d3" = 76.2
  constraints: 1 centre point, 1 coincident, 1 other
  measures "d3" diameter of A0
extrude "Extrusion2" cut sketch "Sketch2" against normal blind 1.27
sketch "Sketch5" plane through (0, 0, 0) normal (1, 0, 0) x (0, 1, 0)
  line L0 (-88.9, -6.35) -> (88.9, -6.35) projected
  line L1 (-63.5, -9.525) -> (-57.15, -9.525)
  line L2 (-57.15, -9.525) -> (-57.15, -6.35)
  line L3 (-63.5, -9.525) -> (-69.85, -9.525)
  line L4 (-69.85, -9.525) -> (-69.85, -6.35)
  line L5 (-57.15, -6.35) -> (-69.85, -6.35)
  line L6 (0, -11.43) -> (0, 1.905) projected
  point P0 (0, 0)
  dimension "d17" = 63.5
  dimension "d18" = 3.175
  dimension "d19" = 12.7
  constraints: 10 end point, 2 collinear, 2 horizontal, 2 perpendicular, 2 point on line
  measures "d17" horizontal distance of L1.start point (0, 0)
  measures "d18" distance of L1.end L2.end
  measures "d19" distance between parallel lines of L4 L2
revolve "Revolution1" add sketch "Sketch5" angle 360 about axis through (0, 0, -10) along (0, 0, 1)
fillet "Fillet1" radius 1.5875 2 edges at (0, 69.85, -9.525) (0, 57.15, -9.525)
equation "\"d0\" = outsideDiameter"
equation "\"d1\" = thickness"
equation "\"d3\" = textRingDiameter"
equation "\"d4\" = textRingDepth"
equation "\"d17\" = glueRingRadius"
equation "\"d18\" = glueRingHeight"
equation "\"d19\" = glueRingWidth"
equation "\"outsideDiameter\" = 177.8"
equation "\"thickness\" = 6.35"
equation "\"glueRingDiameter\" = 127"
equation "\"textRingDiameter\" = 76.2"
equation "\"textRingDepth\" = 1.27"
equation "\"glueRingRadius\" = 0.5 * glueRingDiameter"
equation "\"glueRingWidth\" = 12.7"
equation "\"glueRingHeight\" = 3.175"
body "Solid1"
